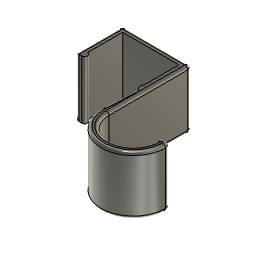
Blind hook v1 (Autodesk Fusion 360 design; units mm, degrees)
Autodesk Fusion 360 part; units mm, degrees
sketch "Sketch1" plane through (0, 0, 0) normal (0, 0, 1) x (1, 0, 0)
  line L0 (14.5, 9) -> (-14.5, 9)
  line L1 (-14.5, 9) -> (-14.5, -9)
  line L2 (14.5, -9) -> (14.5, 9)
  line L3 (14.5, 9) -> (-14.5, -9) construction
  line L4 (-14.5, 9) -> (14.5, -9) construction
  line L5 (17.5, -12) -> (17.5, 12)
  line L6 (17.5, 12) -> (-17.5, 12)
  line L7 (-17.5, 12) -> (-17.5, -12)
  arc A0 (14.5, -9) -> (14.5, -12) centre (16.25, -10.5) ccw
  arc A1 (-14.5, -12) -> (-14.5, -9) centre (-14.5, -10.5) ccw
  line L8 (-17.5, -12) -> (-14.5, -12)
  line L9 (17.5, -12) -> (17.5, -30)
  line L10 (14.5, -12) -> (13.5268, -29.0603)
  arc A2 (17.5, -29.9983) -> (42.5, -30) centre (30, -30) ccw
  arc A3 (13.5268, -29.0603) -> (46.5, -30) centre (30, -30) ccw
  arc A4 (46.5, -30) -> (42.5, -30) centre (44.5, -29.8577) ccw
  dimension "d1" = 29
  dimension "d2" = 18
  dimension "d4" = 25
  dimension "d5" = 33
  constraint horizontal L0
  constraint perpendicular L0 L1
  constraint parallel L1 L2
  constraint coincident L3 origin
  constraint coincident L4 origin
  constraint concentric A2 A3
  constraint coincident A0.end L8
  constraint tangent A1 L8
  constraint tangent L10 A3
  constraint coincident L9 A2.start
  measures "d1" distance of L1.end L2.start
  measures "d2" distance of L0.end L1.end
  measures "d4" diameter of A2
  measures "d5" diameter of A3
extrude "Extrude1" add sketch "Sketch1" along normal blind 30
fillet "Fillet1" radius 1.5 5 edges at (29.9991, -42.5, 30) (17.5, -8.9991, 30) (44.5, -27.8527, 30) (14.0134, -20.5301, 30) (29.5299, -46.4933, 30)
fillet "Fillet2" radius 1.5 5 edges at (17.5, -8.9991, 0) (29.9991, -42.5, 0) (44.5, -27.8527, 0) (14.0134, -20.5301, 0) (29.5299, -46.4933, 0)
fillet "Fillet3" radius 1.5 5 edges at (-0.75, 12, 0) (17.0607, 12, 0.4393) (17.5, 12, 15) (17.0607, 12, 29.5607) (-0.75, 12, 30)
fillet "Fillet4" radius 1.5 1 faces at (-17.5, -4, 19.5)
